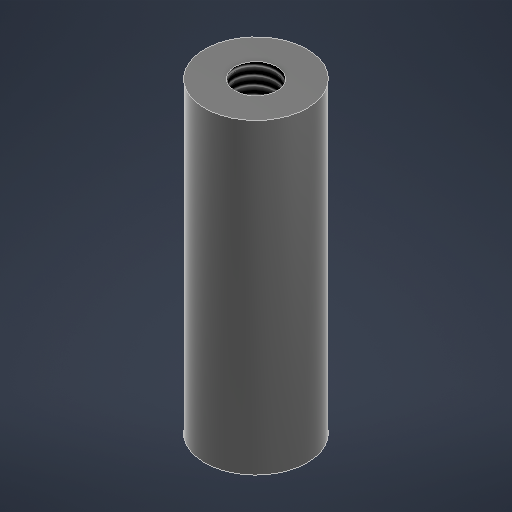
# Autodesk Inventor part: Abstandsbolzen_Kamera
Saved by Autodesk Inventor 2025.2 (Build 292293000, 293)
## iProperties
Created: 2025-03-28
Part Number: Abstandsbolzen_Kamera
Material: Generisch
Document SubType Name: Modeling
Designer: Faabs
Density: 1 g/cm^3
Appearance: Glatt - Schwarz
Author: Faabs
Autodesk Inventor part; units mm, degrees
ref_plane "YZ Plane" through (0, 0, 0) normal (1, 0, 0) x (0, 1, 0)
ref_plane "XZ Plane" through (0, 0, 0) normal (0, 1, 0) x (-1, 0, 0)
ref_plane "XY Plane" through (0, 0, 0) normal (0, 0, 1) x (1, 0, 0)
sketch "Skizze1" plane through (0, 0, 0) normal (0, 0, 1) x (1, 0, 0)
  circle A0 centre (0, 0) radius 3
  dimension "d0" = 6
  constraints: 1 centre point, 1 coincident
  measures "d0" diameter of A0
extrude "Extrusion1" add sketch "Skizze1" along normal mid plane 18
sketch "Skizze3" plane through (0, 0, -9) normal (0, 0, -1) x (-1, 0, 0)
  point P0 (0, 0)
  point P1 (0, 0)
  constraints: 1 coincident
hole "Bohrung2" at (0, 0, -9) direction (0, 0, 1) diameter 2.459 depth 6 tip angle 118 thread size "M3x0.5" class "6H" standard "ISO Metric profile"
mirror "Spiegeln1" about plane through (0, 0, 0) normal (0, 0, 1) of "Bohrung2"
